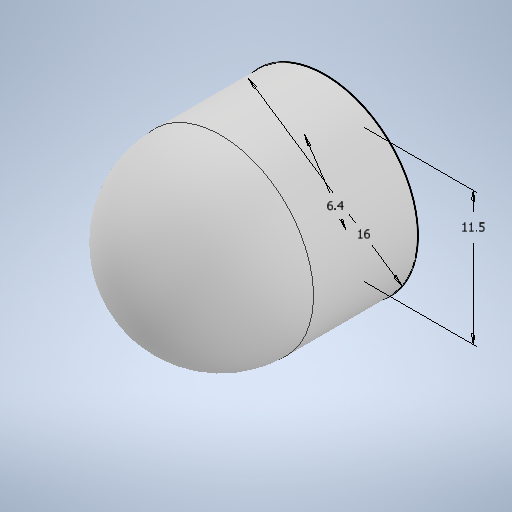
# Autodesk Inventor part: BreakerBoltCover
Saved by Autodesk Inventor 2025.2 (Build 292293000, 293)
## iProperties
Created: 2025-02-25
Part Number: BreakerBoltCover
Material: Generic
Document SubType Name: Modeling
Designer: cutterj
Density: 1 g/cm^3
Appearance: Default
Author: cutterj
Autodesk Inventor part; units mm, degrees
ref_plane "YZ Plane" through (0, 0, 0) normal (1, 0, 0) x (0, 1, 0)
ref_plane "XZ Plane" through (0, 0, 0) normal (0, 1, 0) x (-1, 0, 0)
ref_plane "XY Plane" through (0, 0, 0) normal (0, 0, 1) x (1, 0, 0)
sketch "Sketch1" plane through (0, 0, 0) normal (0, 0, 1) x (1, 0, 0)
  circle A0 centre (0, 0) radius 8
  line L0 (3.3198, 5.75) -> (6.6395, 0)
  line L1 (6.6395, 0) -> (3.3198, -5.75)
  line L2 (3.3198, -5.75) -> (-3.3198, -5.75)
  line L3 (-3.3198, -5.75) -> (-6.6395, 0)
  line L4 (-6.6395, 0) -> (-3.3198, 5.75)
  line L5 (-3.3198, 5.75) -> (3.3198, 5.75)
  circle A1 centre (0, 0) radius 3.2
  dimension "d0" = 16
  dimension "d1" = 11.5
  dimension "d2" = 6.4
  constraints: 12 end point, 4 coincident, 2 centre point, 13 other
  measures "d0" diameter of A0
  measures "d1" distance between parallel lines of L2 L5
  measures "d2" diameter of A1
extrude "Extrusion1" add sketch "Sketch1" along normal blind 17 contours A0 | L0 L1 L2 L3 L4 L5 | A1
fillet "Fillet1" radius 8 1 edges at (-8, 0, 17)
extrude "Extrusion2" cut sketch "Sketch1" along normal blind 13.5 contours A1
extrude "Extrusion3" cut sketch "Sketch1" along normal blind 5.8 contours L0 L1 L2 L3 L4 L5
body "Solid1"
